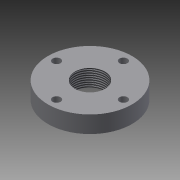
# Autodesk Inventor part: AcmeMountingFlange
Saved by Autodesk Inventor 2013 (Build 170138000, 138)
## iProperties
Created: 2012-12-09
Part Number: AcmeMountingFlange
Material: Generic
Document SubType Name: Modeling
Designer: Istvan
Density: 1 g/cm^3
Author: Istvan
Autodesk Inventor part; units mm, degrees
ref_plane "YZ Plane" through (0, 0, 0) normal (1, 0, 0) x (0, 1, 0)
ref_plane "XZ Plane" through (0, 0, 0) normal (0, 1, 0) x (-1, 0, 0)
ref_plane "XY Plane" through (0, 0, 0) normal (0, 0, 1) x (1, 0, 0)
sketch "Sketch1" plane through (0, 0, 0) normal (0, 1, 0) x (-1, 0, 0)
  circle A0 centre (0, 0) radius 11.9062
  circle A1 centre (0, 0) radius 33.3375
  dimension "d0" = 23.8125
  dimension "d2" = 66.675
  constraints: 2 centre point, 2 coincident
  measures "d0" diameter of A0
  measures "d2" diameter of A1
extrude "Extrusion1" add sketch "Sketch1" along normal blind 13.462
thread "Thread1" size "15/16-16 UN" class "2B" standard "ANSI Unified Screw Threads" full length
sketch "Sketch2" plane through (0, 13.462, 0) normal (0, 1, 0) x (1, 0, 0)
  circle A0 centre (0, 0) radius 11.9062 projected
  circle A1 centre (0, 0) radius 33.3375 projected
  circle A2 centre (0, 0) radius 26.543
  point P0 (0, 26.543)
  point P1 (-26.543, 0)
  point P2 (0, -26.543)
  point P3 (26.543, 0)
  dimension "d7" = 53.086
  constraints: 4 point on circle, 2 horizontal alignment, 2 vertical alignment, 1 centre point, 1 coincident
  measures "d7" diameter of A2
hole "Hole1" at (0, 13.462, -26.543) at (-26.543, 13.462, 0) at (0, 13.462, 26.543) at (26.543, 13.462, 0) direction (0, -1, 0) diameter 6.35 end through all
body "Solid1"
